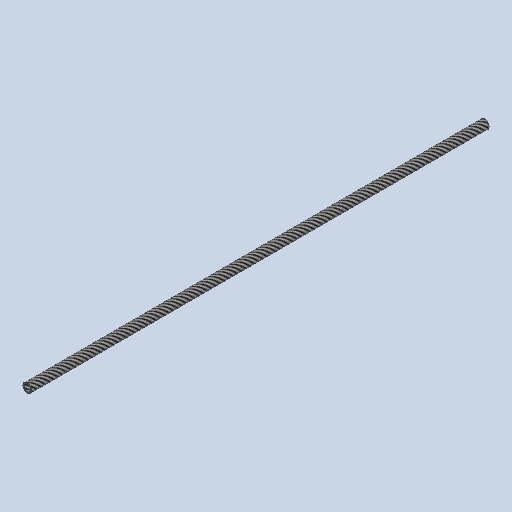
# Autodesk Inventor part: 2P.03.01.04.IM.FlapSpar
Saved by Autodesk Inventor 2025.2 (Build 292293000, 293)
## iProperties
Created: 2025-01-05
Part Number: 2P.03.01.04.IM.FlapSpar
Material: CFRP
Document SubType Name: Modeling
Designer: Imist
Density: 1.43 g/cm^3
Appearance: Carbon Fiber
Author: Imist
Autodesk Inventor part; units mm, degrees
ref_plane "YZ Plane" through (0, 0, 0) normal (1, 0, 0) x (0, 1, 0)
ref_plane "XZ Plane" through (0, 0, 0) normal (0, 1, 0) x (-1, 0, 0)
ref_plane "XY Plane" through (0, 0, 0) normal (0, 0, 1) x (1, 0, 0)
sketch "Sketch1" plane through (0, 0, 0) normal (0, 0, 1) x (1, 0, 0)
  circle A0 centre (-0.0665, -0.0222) radius 3
  circle A1 centre (-0.0665, -0.0222) radius 4
  point P0 (0, 0)
  dimension "d0" = 6
  dimension "d1" = 8
  constraints: 2 centre point, 2 coincident
  measures "d0" diameter of A0
  measures "d1" diameter of A1
extrude "Extrusion1" add sketch "Sketch1" along normal blind 402
body "Solid1"
